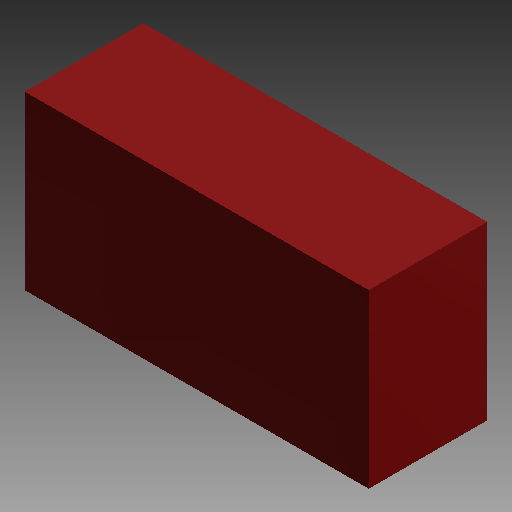
# Autodesk Inventor part: 22r
Saved by Autodesk Inventor 2018.2 (Build 222227000, 227)
## iProperties
Part Number: 22r
Material: Generic
Document SubType Name: Modeling
Designer: autocad
Appearance: R0402, 22r
Author: autocad
Autodesk Inventor part; units mm, degrees
ref_plane "YZ Plane" through (0, 0, 0) normal (1, 0, 0) x (0, 1, 0)
ref_plane "XZ Plane" through (0, 0, 0) normal (0, 1, 0) x (-1, 0, 0)
ref_plane "XY Plane" through (0, 0, 0) normal (0, 0, 1) x (1, 0, 0)
sketch "R0402, 22r_186" plane through (0, 0, 0) normal (0, 0, 1) x (1, 0, 0)
  line L0 (0.508, -0.254) -> (-0.508, -0.254)
  line L1 (-0.508, -0.254) -> (-0.508, 0.254)
  line L2 (-0.508, 0.254) -> (0.508, 0.254)
  line L3 (0.508, 0.254) -> (0.508, -0.254)
  constraints: 8 end point
extrude "Extrusion1" add sketch "R0402, 22r_186" along normal blind 0.35
body "Solid1"
